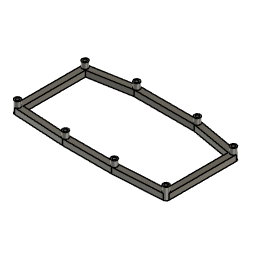
ws22-logic-pcba-release-fixture (Autodesk Fusion 360 design; units mm, degrees)
Autodesk Fusion 360 part; units mm, degrees
note: some values were not read from the file. Set by a fixed rule: the direction of a hole.
sketch "Sketch1" plane through (0, 0, 0) normal (0, 0, 1) x (1, 0, 0)
  circle A0 centre (-76, 32) radius 1.6
  circle A1 centre (-31, 40) radius 1.6
  circle A2 centre (31, 40) radius 1.6
  circle A3 centre (76, 32) radius 1.6
  circle A4 centre (-76, -37) radius 1.6
  circle A5 centre (-24, -40) radius 1.6
  circle A6 centre (26, -40) radius 1.6
  circle A7 centre (76, -37) radius 1.6
  line L0 (-80, 44) -> (80, 44)
  line L1 (80, 44) -> (80, -44)
  line L2 (80, -44) -> (-80, -44)
  line L3 (-80, -44) -> (-80, 44)
  line L4 (80, 44) -> (-80, -44) construction
  dimension "d1" = 3.2
  dimension "d2" = 69
  dimension "d3" = 152
  dimension "d4" = 50
  dimension "d5" = 62
  dimension "d6" = 7
  dimension "d7" = 160
  dimension "d8" = 4
  dimension "d9" = 88
  dimension "d10" = 4
  dimension "d11" = 4
  dimension "d13" = 49
  dimension "d21" = 56
  constraint equal A0 A4
  constraint equal A0 A1
  constraint equal A1 A2
  constraint equal A2 A3
  constraint equal A3 A7
  constraint equal A6 A7
  constraint equal A5 A6
  constraint vertical A3.centre A7.centre
  constraint vertical A0.centre A4.centre
  constraint horizontal A5.centre A6.centre
  constraint horizontal A1.centre A2.centre
  constraint horizontal A0.centre A3.centre
  constraint horizontal A4.centre A7.centre
  constraint horizontal L0
  constraint vertical L1
  constraint horizontal L2
  constraint vertical L3
  constraint midpoint origin L4
  measures "d1" diameter of A0
  measures "d2" distance of A3.centre A7.centre
  measures "d3" distance of A0.centre A3.centre
  measures "d4" distance of A5.centre A6.centre
  measures "d5" distance of A1.centre A2.centre
  measures "d6" distance of A4.centre L2
  measures "d7" distance of L1.end L2.end
  measures "d8" distance of A4.centre L3
  measures "d9" distance of L0.start L2.end
  measures "d10" distance of A5.centre L2
  measures "d11" distance of A1.centre L0
  measures "d13" distance of A2.centre L1
  measures "d21" distance of A5.centre L3
sketch "Sketch2" plane through (0, 0, 0) normal (0, 0, 1) x (1, 0, 0)
  circle A0 centre (-76, 32) radius 1.6 construction
  circle A1 centre (-31, 40) radius 1.6 construction
  circle A2 centre (31, 40) radius 1.6 construction
  circle A3 centre (76, 32) radius 1.6 construction
  circle A4 centre (76, -37) radius 1.6 construction
  circle A5 centre (26, -40) radius 1.6 construction
  circle A6 centre (-24, -40) radius 1.6 construction
  circle A7 centre (-76, -37) radius 1.6 construction
  circle A8 centre (-76, 32) radius 3 construction
  circle A9 centre (-31, 40) radius 3 construction
  circle A10 centre (31, 40) radius 3 construction
  circle A11 centre (76, 32) radius 3 construction
  circle A12 centre (76, -37) radius 3 construction
  circle A13 centre (26, -40) radius 3 construction
  circle A14 centre (-24, -40) radius 3 construction
  circle A15 centre (-76, -37) radius 3 construction
  line L0 (-79, 32) -> (-79, -37)
  arc A16 (-79, -37) -> (-73, -37) centre (-76, -37) ccw
  line L1 (-73, -37) -> (-73, 32)
  arc A17 (-73, 32) -> (-79, 32) centre (-76, 32) ccw
  line L2 (-76, 32) -> (-76, -37) construction
  line L3 (-76.1728, -39.995) -> (-24.1728, -42.995)
  arc A18 (-24.1728, -42.995) -> (-23.8272, -37.005) centre (-24, -40) ccw
  line L4 (-23.8272, -37.005) -> (-75.8272, -34.005)
  arc A19 (-75.8272, -34.005) -> (-76.1728, -39.995) centre (-76, -37) ccw
  line L5 (-76, -37) -> (-24, -40) construction
  line L6 (-75.4749, 29.0463) -> (-30.4749, 37.0463)
  arc A20 (-30.4749, 37.0463) -> (-31.5251, 42.9537) centre (-31, 40) ccw
  line L7 (-31.5251, 42.9537) -> (-76.5251, 34.9537)
  arc A21 (-76.5251, 34.9537) -> (-75.4749, 29.0463) centre (-76, 32) ccw
  line L8 (-76, 32) -> (-31, 40) construction
  line L9 (-31, 37) -> (31, 37)
  arc A22 (31, 37) -> (31, 43) centre (31, 40) ccw
  line L10 (31, 43) -> (-31, 43)
  arc A23 (-31, 43) -> (-31, 37) centre (-31, 40) ccw
  line L11 (-31, 40) -> (31, 40) construction
  line L12 (30.4749, 37.0463) -> (75.4749, 29.0463)
  arc A24 (75.4749, 29.0463) -> (76.5251, 34.9537) centre (76, 32) ccw
  line L13 (76.5251, 34.9537) -> (31.5251, 42.9537)
  arc A25 (31.5251, 42.9537) -> (30.4749, 37.0463) centre (31, 40) ccw
  line L14 (31, 40) -> (76, 32) construction
  line L15 (73, 32) -> (73, -37)
  arc A26 (73, -37) -> (79, -37) centre (76, -37) ccw
  line L16 (79, -37) -> (79, 32)
  arc A27 (79, 32) -> (73, 32) centre (76, 32) ccw
  line L17 (76, 32) -> (76, -37) construction
  line L18 (75.8203, -34.0054) -> (25.8203, -37.0054)
  arc A28 (25.8203, -37.0054) -> (26.1797, -42.9946) centre (26, -40) ccw
  line L19 (26.1797, -42.9946) -> (76.1797, -39.9946)
  arc A29 (76.1797, -39.9946) -> (75.8203, -34.0054) centre (76, -37) ccw
  line L20 (76, -37) -> (26, -40) construction
  line L21 (26, -37) -> (-24, -37)
  arc A30 (-24, -37) -> (-24, -43) centre (-24, -40) ccw
  line L22 (-24, -43) -> (26, -43)
  arc A31 (26, -43) -> (26, -37) centre (26, -40) ccw
  line L23 (26, -40) -> (-24, -40) construction
  dimension "d14" = 6
  constraint concentric A0 A8
  constraint concentric A1 A9
  constraint concentric A2 A10
  constraint concentric A3 A11
  constraint concentric A4 A12
  constraint concentric A5 A13
  constraint concentric A6 A14
  constraint concentric A7 A15
  constraint equal A8 A15
  constraint equal A8 A9
  constraint equal A9 A10
  constraint equal A10 A11
  constraint equal A11 A12
  constraint equal A12 A13
  constraint equal A13 A14
  constraint tangent L0 A16
  constraint tangent A16 L1
  constraint parallel L0 L1
  constraint tangent L1 A17
  constraint tangent L0 A17
  constraint coincident A7.centre A15.centre
  constraint vertical L2
  constraint coincident A0.centre A8.centre
  constraint tangent L3 A18
  constraint tangent A18 L4
  constraint parallel L3 L4
  constraint tangent L4 A19
  constraint tangent L3 A19
  constraint coincident A6.centre A14.centre
  constraint tangent L6 A20
  constraint tangent A20 L7
  constraint parallel L6 L7
  constraint tangent L7 A21
  constraint tangent L6 A21
  constraint coincident A1.centre A9.centre
  constraint tangent L9 A22
  constraint tangent A22 L10
  constraint parallel L9 L10
  constraint tangent L10 A23
  constraint tangent L9 A23
  constraint coincident A2.centre A10.centre
  constraint horizontal L11
  constraint tangent L12 A24
  constraint tangent A24 L13
  constraint parallel L12 L13
  constraint tangent L13 A25
  constraint tangent L12 A25
  constraint coincident A3.centre A11.centre
  constraint tangent L15 A26
  constraint tangent A26 L16
  constraint parallel L15 L16
  constraint tangent L16 A27
  constraint tangent L15 A27
  constraint coincident A4.centre A12.centre
  constraint vertical L17
  constraint tangent L18 A28
  constraint tangent A28 L19
  constraint parallel L18 L19
  constraint tangent L19 A29
  constraint tangent L18 A29
  constraint coincident A5.centre A13.centre
  constraint tangent L21 A30
  constraint tangent A30 L22
  constraint parallel L21 L22
  constraint tangent L22 A31
  constraint tangent L21 A31
  constraint horizontal L23
  constraint coincident A14 L21.end
  constraint coincident A14 A18.end
  constraint coincident A13 L18.end
  constraint coincident A12 L15.end
  constraint coincident A11 L12.end
  constraint coincident A10 L9.end
  constraint coincident A9 L6.end
  constraint coincident A8 L1.end
  measures "d14" diameter of A8
extrude "Extrude1" add sketch "Sketch2" along normal blind 6 contours L0 L1 L4 A19 L6 A21 | L1 A17 L6 A21 | A16 L1 L4 A19 | L1 A17 L6 L7 L9 A23 | A16 L1 L3 L4 L21 A30 | L6 A20 L9 A23 | A18 L4 L21 A30 | L6 A20 L9 L10 L12 A25 | A18 L4 L18 A28 L21 L22 | L9 A22 L12 A25 | L9 A22 L12 L13 L15 A27 | L18 A28 L21 A31 | L15 A26 L18 L19 L21 A31 | L12 A24 L15 A27 | L12 A24 L15 L16 L18 A29 | L15 A26 L18 A29
sketch "Sketch3" plane through (0, 0, 0) normal (0, 0, -1) x (1, 0, 0)
  circle A0 centre (-76, 37) radius 3
  circle A1 centre (-24, 40) radius 3
  circle A2 centre (26, 40) radius 3
  circle A3 centre (76, 37) radius 3
  circle A4 centre (76, -32) radius 3
  circle A5 centre (31, -40) radius 3
  circle A6 centre (-31, -40) radius 3
  circle A7 centre (-76, -32) radius 3
extrude "Extrude2" add sketch "Sketch3" against normal blind 12
hole "Hole1" at (76, 32, 0) at (31, 40, 0) at (-31, 40, 0) at (-76, 32, 0) at (-76, -37, 0) at (-24, -40, 0) at (26, -40, 0) at (76, -37, 0) direction (0, 0, 1) diameter 3.2 end through all
equation "d6 = 5.4 mm + ( ( 3.2 / 2 ) * 1 mm )"
equation "d8 = 2.4 mm + ( ( 3.2 / 2 ) * 1 mm )"
equation "d10 = 2.4 mm + ( ( 3.2 / 2 ) * 1 mm )"
equation "d11 = 2.4 mm + ( ( 3.2 / 2 ) * 1 mm )"
equation "d13 = 47.4 mm + ( ( 3.2 / 2 ) * 1 mm )"
equation "d21 = 54.4 mm + ( ( 3.2 / 2 ) * 1 mm )"
named bodies: "WS22 logic board release fixture"
